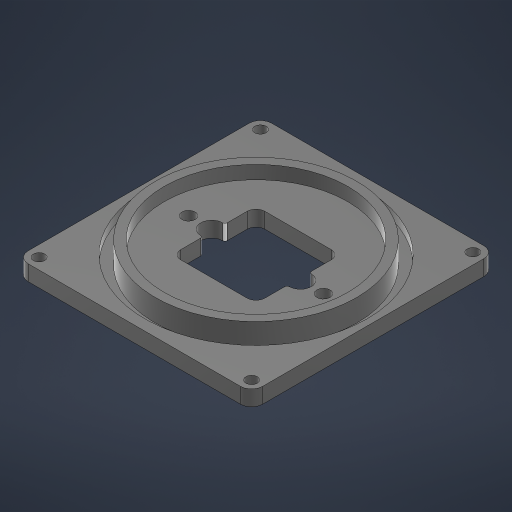
# Autodesk Inventor part: Camera_Mount
Saved by Autodesk Inventor 2024.2 (Build 282272000, 272)
## iProperties
Created: 2024-01-10
Part Number: Camera_Mount
Material: 一般
Document SubType Name: Modeling
Designer: Hanaoka
Density: 1 g/cm^3
Appearance: 既定
Author: Hanaoka
Autodesk Inventor part; units mm, degrees
ref_plane "YZ Plane" through (0, 0, 0) normal (1, 0, 0) x (0, 1, 0)
ref_plane "XZ Plane" through (0, 0, 0) normal (0, 1, 0) x (-1, 0, 0)
ref_plane "作業平面1" through (-1.8524, -8.2893, -39.454) normal (0, 1, 0) x (1, 0, 0)
sketch "スケッチ1" plane through (-1.8524, -8.2893, -39.454) normal (0, 1, 0) x (1, 0, 0)
  line L0 (9.655, 16.755) -> (9.655, 15.8775) projected
  arc A0 (6.855, 15.8775) -> (9.655, 15.8775) centre (8.255, 8.255) ccw projected
  line L1 (6.855, 15.8775) -> (6.855, 16.755) projected
  line L2 (6.855, 16.755) -> (0.755, 16.755) projected
  arc A1 (0.755, 16.755) -> (-0.245, 15.755) centre (0.755, 15.755) ccw projected
  line L3 (-0.245, 15.755) -> (-0.245, 10.155) projected
  line L4 (-0.245, 10.155) -> (-1.745, 10.155) projected
  arc A2 (-1.745, 10.155) -> (-1.745, 6.355) centre (-1.745, 8.255) ccw projected
  line L5 (-1.745, 6.355) -> (-0.245, 6.355) projected
  line L6 (-0.245, 6.355) -> (-0.245, 0.755) projected
  arc A3 (-0.245, 0.755) -> (0.755, -0.245) centre (0.755, 0.755) ccw projected
  line L7 (0.755, -0.245) -> (15.755, -0.245) projected
  arc A4 (15.755, -0.245) -> (16.755, 0.755) centre (15.755, 0.755) ccw projected
  line L8 (16.755, 0.755) -> (16.755, 6.355) projected
  line L9 (16.755, 6.355) -> (18.255, 6.355) projected
  arc A5 (18.255, 6.355) -> (18.255, 10.155) centre (18.255, 8.255) ccw projected
  line L10 (18.255, 10.155) -> (16.755, 10.155) projected
  line L11 (16.755, 10.155) -> (16.755, 15.755) projected
  arc A6 (16.755, 15.755) -> (15.755, 16.755) centre (15.755, 15.755) ccw projected
  line L12 (15.755, 16.755) -> (9.655, 16.755) projected
  circle A7 centre (-1.745, 8.255) radius 0.9 projected
  circle A8 centre (18.255, 8.255) radius 0.9 projected
  line L13 (-15.745, -19.245) -> (32.255, -19.245)
  line L14 (34.755, -16.745) -> (34.755, 33.255)
  line L15 (32.255, 35.755) -> (-15.745, 35.755)
  line L16 (-18.245, 33.255) -> (-18.245, -16.745)
  line L17 (-18.245, -19.245) -> (34.755, 35.755) construction
  line L18 (34.755, -19.245) -> (-18.245, 35.755) construction
  arc A9 (-15.745, 35.755) -> (-18.245, 33.255) centre (-15.745, 33.255) ccw
  arc A10 (34.755, 33.255) -> (32.255, 35.755) centre (32.255, 33.255) ccw
  arc A11 (32.255, -19.245) -> (34.755, -16.745) centre (32.255, -16.745) ccw
  arc A12 (-18.245, -16.745) -> (-15.745, -19.245) centre (-15.745, -16.745) ccw
  circle A13 centre (-15.745, 33.255) radius 1.3
  circle A14 centre (32.255, 33.255) radius 1.3
  circle A15 centre (32.255, -16.745) radius 1.3
  circle A16 centre (-15.745, -16.745) radius 1.3
  line L19 (32.255, -16.745) -> (-15.745, -16.745) construction
  line L20 (-15.745, -16.745) -> (-15.745, 33.255) construction
  line L21 (-15.745, 33.255) -> (32.255, 33.255) construction
  line L22 (32.255, 33.255) -> (32.255, -16.745) construction
  line L23 (32.255, -16.745) -> (-15.745, 33.255) construction
  line L24 (-15.745, -16.745) -> (32.255, 33.255) construction
  line L25 (6.855, 16.755) -> (9.655, 16.755)
  circle A17 centre (-6.985, 8.255) radius 1.5 projected
  circle A18 centre (18.26, 8.26) radius 1.27 projected
  circle A19 centre (23.495, 8.255) radius 1.5 projected
  arc A20 (-1.745, 10.755) -> (-1.745, 5.755) centre (-1.745, 8.255) ccw
  arc A21 (18.26, 5.76) -> (18.26, 10.76) centre (18.26, 8.26) ccw
  arc A22 (17.755, 15.755) -> (15.755, 17.755) centre (15.755, 15.755) ccw
  arc A23 (15.755, -1.245) -> (17.755, 0.755) centre (15.755, 0.755) ccw
  arc A24 (-1.245, 0.755) -> (0.755, -1.245) centre (0.755, 0.755) ccw
  arc A25 (0.755, 17.755) -> (-1.245, 15.755) centre (0.755, 15.755) ccw
  line L26 (0.755, 17.755) -> (15.755, 17.755)
  line L27 (17.755, 15.755) -> (17.755, 10.76)
  line L28 (17.755, 10.76) -> (18.26, 10.76)
  line L29 (17.755, 0.755) -> (17.755, 5.76)
  line L30 (17.755, 5.76) -> (18.26, 5.76)
  line L31 (15.755, -1.245) -> (0.755, -1.245)
  line L32 (-1.245, 0.755) -> (-1.245, 5.755)
  line L33 (-1.245, 5.755) -> (-1.745, 5.755)
  line L34 (-1.745, 10.755) -> (-1.245, 10.755)
  line L35 (-1.245, 10.755) -> (-1.245, 15.755)
  point P0 (1.8524, -39.454)
  dimension "d2" = 2.5
  dimension "d3" = 2.6
  dimension "d4" = 50
  dimension "d5" = 48
  dimension "d15" = 2.5
  dimension "d16" = 2
  constraints: 46 end point, 22 point on circle, 20 tangent, 16 parallel, 14 centre point, 10 coincident, 9 point on line, 8 equal radius, 4 horizontal, 4 midpoint, 3 perpendicular
  measures "d2" radius of A9
  measures "d3" diameter of A14
  measures "d4" distance of L19.end L20.end
  measures "d5" distance of L20.end L21.end
  measures "d15" radius of A20
  measures "d16" radius of A25
extrude "押し出し1" add sketch "スケッチ1" along normal blind 3.5 contours A12 L16 A9 L15 A10 L14 A11 L13
sketch "スケッチ2" plane through (-1.8524, -4.7893, -39.454) normal (0, 1, 0) x (1, 0, 0)
  arc A0 (32.255, -19.245) -> (34.755, -16.745) centre (32.255, -16.745) ccw projected
  line L0 (34.755, -16.745) -> (34.755, 33.255) projected
  arc A1 (34.755, 33.255) -> (32.255, 35.755) centre (32.255, 33.255) ccw projected
  line L1 (32.255, 35.755) -> (-15.745, 35.755) projected
  arc A2 (-15.745, 35.755) -> (-18.245, 33.255) centre (-15.745, 33.255) ccw projected
  line L2 (-18.245, 33.255) -> (-18.245, -16.745) projected
  arc A3 (-18.245, -16.745) -> (-15.745, -19.245) centre (-15.745, -16.745) ccw projected
  line L3 (-15.745, -19.245) -> (32.255, -19.245) projected
  circle A4 centre (-15.745, -16.745) radius 1.3 projected
  circle A5 centre (32.255, -16.745) radius 1.3 projected
  circle A6 centre (32.255, 33.255) radius 1.3 projected
  circle A7 centre (-15.745, 33.255) radius 1.3 projected
  circle A8 centre (8.255, 8.255) radius 25.1
  circle A9 centre (8.255, 8.255) radius 22.75
  circle A10 centre (8.255, 8.255) radius 20.75
  point P0 (1.8524, -39.454)
  dimension "d8" = 50.2
  dimension "d9" = 45.5
  dimension "d10" = 2
  constraints: 3 centre point, 2 coincident
  measures "d8" diameter of A8
  measures "d9" diameter of A9
  measures "d10" radial gap between concentric circles of A9 A10
extrude "押し出し2" add sketch "スケッチ2" along normal blind 3 contours A9
extrude "押し出し3" cut sketch "スケッチ2" against normal blind 2 contours A8
fillet "フィレット1" radius 0.5 4 edges at (-3.0974, -6.5393, -50.209) (-3.0974, -6.5393, -45.209) (15.9026, -6.5393, -50.214) (15.9026, -6.5393, -45.214)
